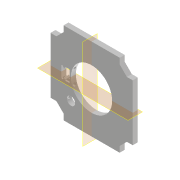
# Autodesk Inventor part: 20_Cube_Insert_lineartranlator_mgn7_base_v3
Saved by Autodesk Inventor 2022 (Build 260153000, 153)
## iProperties
Created: 2019-07-01
Part Number: 20_Cube_Insert_lineartranlator_mgn7_base_v3
Material: Generic
Document SubType Name: Modeling
Designer: diederichbenedict
Density: 1 g/cm^3
Appearance: Default
Author: diederichbenedict
Autodesk Inventor part; units mm, degrees
ref_plane "YZ Plane" through (0, 0, 0) normal (1, 0, 0) x (0, 1, 0)
ref_plane "XZ Plane" through (0, 0, 0) normal (0, 1, 0) x (-1, 0, 0)
ref_plane "Work Plane1" through (0, 0, 10) normal (0, 0, 1) x (1, 0, 0)
sketch "Sketch1" plane through (0, 0, 10) normal (0, 0, 1) x (1, 0, 0)
  line L0 (-4.0299, -0.3538) -> (-2.2322, 1.4439) construction
  arc A0 (-1.4439, 2.2322) -> (-2.2322, 1.4439) centre (-0.9299, 0.9299) ccw construction
  line L1 (-1.4439, 2.2322) -> (0.3538, 4.0299) construction
  line L2 (-37.8299, 42.8299) -> (-37.8299, 37.8299) construction
  line L3 (-37.8299, 37.8299) -> (-42.9208, 37.8299) construction
  line L4 (-37.8299, 42.2137) -> (-37.8299, 45.8299) construction
  line L5 (-37.8299, 45.8299) -> (-4.0299, 45.8299) construction
  line L6 (-4.0299, 45.8299) -> (-4.0299, 42.2137) construction
  line L7 (-4.0299, 4.0299) -> (0.3538, 4.0299) projected
  circle A1 centre (-20.9299, 20.9299) radius 17.5 projected
  line L8 (-20.9299, 58.9723) -> (17.1124, 20.9299) construction
  line L9 (17.1124, 20.9299) -> (-20.9299, -17.1124) construction
  line L10 (-20.9299, -17.1124) -> (-58.9723, 20.9299) construction
  line L11 (-58.9723, 20.9299) -> (-20.9299, 58.9723) construction
  line L12 (-20.9299, 58.9723) -> (-20.9299, -17.1124) construction
  line L13 (17.1124, 20.9299) -> (-58.9723, 20.9299) construction
  line L14 (-20.9299, 58.9723) -> (32.8701, 58.9723) construction
  line L15 (-43.4299, 43.4299) -> (1.5701, 43.4299) construction
  line L16 (1.5701, 43.4299) -> (1.5701, -1.5701) construction
  line L17 (1.5701, -1.5701) -> (-43.4299, -1.5701) construction
  line L18 (-43.4299, -1.5701) -> (-43.4299, 43.4299) construction
  line L19 (-43.4299, 43.4299) -> (1.5701, -1.5701) construction
  line L20 (1.5701, 43.4299) -> (-43.4299, -1.5701) construction
  line L21 (-43.4299, 5.3876) -> (-43.4299, 36.4723)
  line L22 (-43.4299, 36.4723) -> (-36.4723, 43.4299)
  line L23 (-36.4723, 43.4299) -> (-5.3876, 43.4299)
  line L24 (-5.3876, 43.4299) -> (1.5701, 36.4723)
  line L25 (1.5701, 36.4723) -> (1.5701, 5.3876)
  line L26 (1.5701, 5.3876) -> (-5.3876, -1.5701)
  line L27 (-5.3876, -1.5701) -> (-36.4723, -1.5701)
  line L28 (-36.4723, -1.5701) -> (-43.4299, 5.3876)
  line L29 (-4.0299, 42.2137) -> (-37.8299, 42.2137) projected
  line L30 (-4.0299, -0.3538) -> (-4.0299, 4.0299) projected
  circle A2 centre (-20.9299, 20.9299) radius 1.5
  line L31 (-10.9299, 10.9299) -> (-30.9299, 10.9299) construction
  line L32 (-30.9299, 10.9299) -> (-30.9299, 30.9299) construction
  line L33 (-30.9299, 30.9299) -> (-10.9299, 30.9299) construction
  line L34 (-10.9299, 30.9299) -> (-10.9299, 10.9299) construction
  line L35 (-10.9299, 10.9299) -> (-30.9299, 30.9299) construction
  line L36 (-30.9299, 10.9299) -> (-10.9299, 30.9299) construction
  circle A3 centre (-30.9299, 30.9299) radius 1.4
  circle A4 centre (-30.9299, 10.9299) radius 1.4
  circle A5 centre (-10.9299, 10.9299) radius 1.4
  line L37 (-45.8299, 37.8299) -> (-42.0723, 37.8299) construction
  line L38 (-42.1723, 37.7299) -> (-45.8299, 37.7299)
  line L39 (-45.8299, 37.7299) -> (-45.8299, 4.1299)
  line L40 (-45.8299, 4.1299) -> (-42.1723, 4.1299)
  line L41 (-42.1723, 4.1299) -> (-42.1723, 37.7299)
  line L42 (-45.8299, 4.0299) -> (-42.0723, 4.0299) construction
  line L43 (-45.8299, 37.8299) -> (-42.0723, 37.8299) projected
  line L44 (-37.7299, 45.8299) -> (-4.1299, 45.8299)
  line L45 (-4.1299, 45.8299) -> (-4.1299, 42.1723)
  line L46 (-4.1299, 42.1723) -> (-37.7299, 42.1723)
  line L47 (-37.7299, 42.1723) -> (-37.7299, 45.8299)
  line L48 (0.4701, 37.8299) -> (0.4701, 4.0299) construction
  line L49 (0.4701, 4.0299) -> (3.9701, 4.0299) construction
  line L50 (3.9701, 37.8299) -> (3.9701, 4.0299) construction
  line L51 (0.4701, 37.8299) -> (3.9701, 37.8299) construction
  line L52 (-45.8299, -3.9701) -> (-4.0299, -3.9701) construction
  line L53 (0.3124, 37.7299) -> (3.9701, 37.7299)
  line L54 (3.9701, 37.7299) -> (3.9701, 4.1299)
  line L55 (3.9701, 4.1299) -> (0.3124, 4.1299)
  line L56 (0.3124, 4.1299) -> (0.3124, 37.7299)
  line L57 (-4.1713, -0.3538) -> (-37.7299, -0.3538)
  line L58 (-37.7299, -0.3538) -> (-37.7299, -3.9701)
  line L59 (-37.7299, -3.9701) -> (-4.1713, -3.9701)
  line L60 (-4.1713, -3.9701) -> (-4.1713, -0.3538)
  point P0 (-37.8299, 4.0299)
  dimension "d18" = 53.8
  dimension "d19" = 45
  dimension "d20" = 53.8
  dimension "d21" = 45
  dimension "d22" = 45
  dimension "d30" = 20
  dimension "d31" = 20
  dimension "d32" = 2.8
  dimension "d33" = 2.8
  dimension "d34" = 2.8
  dimension "d35" = 3
  dimension "d36" = 0.1
  dimension "d37" = 0.1
  dimension "d38" = 0.1
  dimension "d39" = 0.1
  constraints: 86 end point, 21 point on line, 14 parallel, 8 perpendicular, 7 horizontal, 7 midpoint, 4 centre point, 4 coincident, 1 equal length
  measures "d18" distance of L8.start L8.end
  measures "d19" angle of L8 L14
  measures "d20" distance of L8.end L9.end
  measures "d21" distance of L16.end L17.end
  measures "d22" distance of L15.end L16.end
  measures "d30" distance of L32.end L33.end
  measures "d31" distance of L31.end L32.end
  measures "d32" diameter of A3
  measures "d33" diameter of A4
  measures "d34" diameter of A5
  measures "d35" diameter of A2
  measures "d36" distance between parallel lines of L38 L43
  measures "d37" distance between parallel lines of L40 L42
  measures "d38" distance between parallel lines of L45 L6
  measures "d39" distance between parallel lines of L4 L47
extrude "Extrusion1" add sketch "Sketch1" along normal blind 3 contours L30 L26 L57 L28 L41 L22 L46 L24 L56 L7 | L7 L26 L30 | L56 L24 L25 L26 | L26 L25 L24 L53 L54 L55 | L60 L59 L58 L57 L28 L27 L26 | L26 L27 L28 L57 | L46 L22 L29 L24 | L24 L29 L45 | L40 L39 L38 L22 L21 L28 | L28 L21 L22 L41 | L29 L22 L23 L24 | L24 L23 L22 L29 L47 L44 L45 | L47 L29 L22 | A1 | A2 | A3 | A4 | A5
sketch "Skizze4" plane through (0, 0, 13) normal (0, 0, 1) x (1, 0, 0)
  line L0 (-37.7299, 42.1723) -> (-42.1723, 37.7299) projected
  line L1 (-42.1723, 37.7299) -> (-45.8299, 37.7299) projected
  line L2 (-45.8299, 37.7299) -> (-45.8299, 4.1299) construction
  line L3 (-45.8299, 4.1299) -> (-42.1723, 4.1299) projected
  line L4 (-42.1723, 4.1299) -> (-37.6885, -0.3538) projected
  line L5 (-37.6885, -0.3538) -> (-37.7299, -0.3538) projected
  line L6 (-37.7299, -0.3538) -> (-37.7299, -3.9701) projected
  line L7 (-37.7299, -3.9701) -> (-4.1713, -3.9701) construction
  line L8 (-4.1713, -3.9701) -> (-4.1713, -0.3538) projected
  line L9 (-4.1713, -0.3538) -> (0.3124, 4.1299) projected
  line L10 (0.3124, 4.1299) -> (3.9701, 4.1299) projected
  line L11 (3.9701, 4.1299) -> (3.9701, 37.7299) construction
  line L12 (3.9701, 37.7299) -> (0.3124, 37.7299) projected
  line L13 (0.3124, 37.7299) -> (-4.1299, 42.1723) projected
  line L14 (-4.1299, 42.1723) -> (-4.1299, 45.8299) projected
  line L15 (-4.1299, 45.8299) -> (-37.7299, 45.8299) construction
  line L16 (-37.7299, 45.8299) -> (-37.7299, 42.1723) projected
  line L17 (-37.9299, 46.0299) -> (-3.9299, 46.0299) construction
  line L18 (-3.9299, 46.0299) -> (-3.9299, 42.2551)
  line L19 (-3.9299, 42.2551) -> (0.3953, 37.9299)
  line L20 (0.3953, 37.9299) -> (4.1701, 37.9299)
  line L21 (4.1701, 37.9299) -> (4.1701, 3.9299) construction
  line L22 (4.1701, 3.9299) -> (0.3953, 3.9299)
  line L23 (0.3953, 3.9299) -> (-3.9713, -0.4367)
  line L24 (-3.9713, -0.4367) -> (-3.9713, -4.1701)
  line L25 (-3.9713, -4.1701) -> (-37.9299, -4.1701) construction
  line L26 (-37.9299, -4.1701) -> (-37.9299, -0.3953)
  line L27 (-37.9299, -0.3953) -> (-42.2551, 3.9299)
  line L28 (-42.2551, 3.9299) -> (-46.0299, 3.9299)
  line L29 (-46.0299, 3.9299) -> (-46.0299, 37.9299) construction
  line L30 (-46.0299, 37.9299) -> (-42.2551, 37.9299)
  line L31 (-42.2551, 37.9299) -> (-37.9299, 42.2551)
  line L32 (-37.9299, 42.2551) -> (-37.9299, 46.0299)
  line L33 (-45.8299, 37.7299) -> (-45.8299, 37.9299)
  line L34 (-4.1299, 45.8299) -> (-37.7299, 45.8299) projected
  line L35 (-37.7299, 45.8299) -> (-37.9299, 45.8299)
  line L36 (-4.1299, 45.8299) -> (-3.9299, 45.8299)
  line L37 (3.9701, 37.7299) -> (3.9701, 37.9299)
  line L38 (3.9701, 4.1299) -> (3.9701, 37.7299) projected
  line L39 (3.9701, 4.1299) -> (3.9701, 3.9299)
  line L40 (-4.1713, -3.9701) -> (-3.9713, -3.9701)
  line L41 (-37.7299, -3.9701) -> (-37.9299, -3.9701)
  line L42 (-45.8299, 4.1299) -> (-45.8299, 3.9299)
  point P0 (0, 0)
  dimension "d40" = 0.2
  constraints: 48 end point, 12 point on line, 4 perpendicular, 15 other
  measures "d40" distance between parallel lines of L15 L17
extrude "IM_offset" add sketch "Skizze4" against normal up to surface (3 mm away)
ref_plane "Arbeitsebene5" through (-20.9299, 3.9299, 10) normal (1, 0, 0) x (0, 0, -1)
ref_plane "Arbeitsebene6" through (-37.9299, 20.9299, 10) normal (0, 1, 0) x (1, 0, 0)
sketch "Skizze25" plane through (0, 0, 13) normal (0, 0, 1) x (1, 0, 0)
  arc A0 (-37.9299, 18.0899) -> (-38.4737, 17.4299) centre (-37.6799, 17.3299) ccw projected
  line L0 (-37.9299, 18.0899) -> (-37.9299, 18.5899) projected
  line L1 (-37.9299, 18.5899) -> (-37.4299, 18.5899) projected
  line L2 (-37.4299, 18.5899) -> (-37.4299, 18.0899) projected
  arc A1 (-36.8862, 17.4299) -> (-37.4299, 18.0899) centre (-37.6799, 17.3299) ccw projected
  line L3 (-36.8862, 17.4299) -> (-34.5799, 17.4299) projected
  line L4 (-34.5799, 17.4299) -> (-34.3799, 17.6299) projected
  line L5 (-34.3799, 17.6299) -> (-34.3799, 24.2299) projected
  line L6 (-34.3799, 24.2299) -> (-34.5799, 24.4299) projected
  line L7 (-34.5799, 24.4299) -> (-36.8862, 24.4299) projected
  arc A2 (-37.4299, 23.77) -> (-36.8862, 24.4299) centre (-37.6799, 24.5299) ccw projected
  line L8 (-37.4299, 23.77) -> (-37.4299, 23.27) projected
  line L9 (-37.4299, 23.27) -> (-37.9299, 23.27) projected
  line L10 (-37.9299, 23.27) -> (-37.9299, 23.77) projected
  arc A3 (-38.4737, 24.4299) -> (-37.9299, 23.77) centre (-37.6799, 24.5299) ccw projected
  line L11 (-38.4737, 24.4299) -> (-38.9799, 24.4299) projected
  line L12 (-38.9799, 24.4299) -> (-39.1799, 24.2299) projected
  line L13 (-39.1799, 24.2299) -> (-39.1799, 17.6299) projected
  line L14 (-39.1799, 17.6299) -> (-38.9799, 17.4299) projected
  line L15 (-38.9799, 17.4299) -> (-38.4737, 17.4299) projected
  line L16 (-34.2799, 24.2713) -> (-34.2799, 17.5885)
  line L17 (-34.2799, 17.5885) -> (-34.5385, 17.3299)
  line L18 (-34.5385, 17.3299) -> (-36.9799, 17.3299)
  arc A4 (-36.9799, 17.3299) -> (-37.5299, 18.0137) centre (-37.6799, 17.3299) ccw
  line L19 (-37.5299, 18.0137) -> (-37.5299, 18.4899)
  line L20 (-37.5299, 18.4899) -> (-37.8299, 18.4899)
  line L21 (-37.8299, 18.4899) -> (-37.8299, 18.0137)
  arc A5 (-37.8299, 18.0137) -> (-38.3799, 17.3299) centre (-37.6799, 17.3299) ccw
  line L22 (-38.3799, 17.3299) -> (-39.0213, 17.3299)
  line L23 (-39.0213, 17.3299) -> (-39.2799, 17.5885)
  line L24 (-39.2799, 17.5885) -> (-39.2799, 24.2713)
  line L25 (-39.2799, 24.2713) -> (-39.0213, 24.5299)
  line L26 (-39.0213, 24.5299) -> (-38.3799, 24.5299)
  arc A6 (-38.3799, 24.5299) -> (-37.8299, 23.8462) centre (-37.6799, 24.5299) ccw
  line L27 (-37.8299, 23.8462) -> (-37.8299, 23.37)
  line L28 (-37.8299, 23.37) -> (-37.5299, 23.37)
  line L29 (-37.5299, 23.37) -> (-37.5299, 23.8462)
  arc A7 (-37.5299, 23.8462) -> (-36.9799, 24.5299) centre (-37.6799, 24.5299) ccw
  line L30 (-36.9799, 24.5299) -> (-34.5385, 24.5299)
  line L31 (-34.5385, 24.5299) -> (-34.2799, 24.2713)
  circle A8 centre (-21.0099, 20.9299) radius 10.125 projected
  circle A9 centre (-21.0099, 20.9299) radius 12.5
  point P0 (0, 0)
  dimension "d150" = 0.1
  dimension "d151" = 25
  constraints: 32 end point, 8 point on circle, 5 centre point, 1 coincident, 19 other
  measures "d150" distance between parallel lines of L5 L16
  measures "d151" diameter of A9
extrude "Extrusion21" cut sketch "Skizze25" against normal blind 3 contours A0 L15 L14 L13 L12 L11 A3 L10 L9 L8 A2 L7 L6 L5 L4 L3 A1 L2 L1 L0 | L16 L17 L18 A4 L19 L20 L21 A5 L22 L23 L24 L25 L26 A6 L27 L28 L29 A7 L30 L31 | A8 | A9
sketch "Skizze26" plane through (-45.8299, 3.9299, 10) normal (-1, 0, 0) x (0, 0, 1)
  line L0 (0, 0) -> (0, 34) projected
  line L1 (3, 0) -> (0, 0) projected
  line L2 (3, 34) -> (3, 0) projected
  line L3 (3, 34) -> (0, 34) projected
  line L4 (3, 29.5) -> (0, 29.5) projected
  circle A0 centre (1.5, 29.5) radius 0.9
  line L5 (3, 4.5) -> (0, 4.5) projected
  circle A1 centre (1.5, 4.5) radius 0.9
  line L6 (36.97, 20.3) -> (-3.03, 20.3) projected
  line L7 (36.97, 13.7) -> (-3.03, 13.7) projected
  circle A2 centre (1.5, 21.2) radius 0.9
  circle A3 centre (1.5, 12.8) radius 0.9
  point P0 (-10, -3.9299)
  dimension "d154" = 1.8
  dimension "d155" = 1.8
  dimension "d158" = 1.8
  dimension "d159" = 1.8
  constraints: 4 centre point, 2 midpoint, 2 tangent
  measures "d154" diameter of A0
  measures "d155" diameter of A1
  measures "d158" diameter of A2
  measures "d159" diameter of A3
extrude "Extrusion22" cut sketch "Skizze26" against normal blind 15 contours A3 | A1 L5 | L5 A1 | A2 | A0 L4 | L4 A0
sketch "Skizze27" plane through (0, 0, 10) normal (0, 0, -1) x (-1, 0, 0)
  arc A0 (36.9799, 24.5299) -> (37.5299, 23.8462) centre (37.6799, 24.5299) ccw projected
  line L0 (37.5299, 23.8462) -> (37.5299, 23.37) projected
  line L1 (37.5299, 23.37) -> (37.8299, 23.37) projected
  line L2 (37.8299, 23.37) -> (37.8299, 23.8462) projected
  arc A1 (37.8299, 23.8462) -> (38.3799, 24.5299) centre (37.6799, 24.5299) ccw projected
  line L3 (38.3799, 24.5299) -> (39.0213, 24.5299) projected
  line L4 (39.0213, 24.5299) -> (39.2799, 24.2713) projected
  line L5 (39.2799, 24.2713) -> (39.2799, 17.5885) projected
  line L6 (39.2799, 17.5885) -> (39.0213, 17.3299) projected
  line L7 (39.0213, 17.3299) -> (38.3799, 17.3299) projected
  arc A2 (38.3799, 17.3299) -> (37.8299, 18.0137) centre (37.6799, 17.3299) ccw projected
  line L8 (37.8299, 18.0137) -> (37.8299, 18.4899) projected
  line L9 (37.8299, 18.4899) -> (37.5299, 18.4899) projected
  line L10 (37.5299, 18.4899) -> (37.5299, 18.0137) projected
  arc A3 (37.5299, 18.0137) -> (36.9799, 17.3299) centre (37.6799, 17.3299) ccw projected
  line L11 (36.9799, 17.3299) -> (34.5385, 17.3299) projected
  line L12 (34.5385, 17.3299) -> (34.2799, 17.5885) projected
  line L13 (34.2799, 17.5885) -> (34.2799, 24.2713) projected
  line L14 (34.2799, 24.2713) -> (34.5385, 24.5299) projected
  line L15 (34.5385, 24.5299) -> (36.9799, 24.5299) projected
  circle A4 centre (21.0099, 20.9299) radius 12.5 projected
  line L16 (3.9713, -3.9701) -> (37.9299, -3.9701) projected
  line L17 (37.9299, -3.9701) -> (37.9299, -0.3953) projected
  line L18 (37.9299, -0.3953) -> (42.2551, 3.9299) projected
  line L19 (42.2551, 3.9299) -> (45.8299, 3.9299) projected
  line L20 (45.8299, 3.9299) -> (45.8299, 37.9299) projected
  line L21 (45.8299, 37.9299) -> (42.2551, 37.9299) projected
  line L22 (42.2551, 37.9299) -> (37.9299, 42.2551) projected
  line L23 (37.9299, 42.2551) -> (37.9299, 45.8299) projected
  line L24 (37.9299, 45.8299) -> (3.9299, 45.8299) projected
  line L25 (3.9299, 45.8299) -> (3.9299, 42.2551) projected
  line L26 (3.9299, 42.2551) -> (-0.3953, 37.9299) projected
  line L27 (-0.3953, 37.9299) -> (-3.9701, 37.9299) projected
  line L28 (-3.9701, 37.9299) -> (-3.9701, 3.9299) projected
  line L29 (-3.9701, 3.9299) -> (-0.3953, 3.9299) projected
  line L30 (-0.3953, 3.9299) -> (3.9713, -0.4367) projected
  line L31 (3.9713, -0.4367) -> (3.9713, -3.9701) projected
  line L32 (37.9799, 3.9599) -> (37.9799, 43.7799) projected
  line L33 (37.9799, 3.9599) -> (3.8799, 3.9599) projected
  circle A5 centre (33.4322, 8.4277) radius 3
  circle A6 centre (33.4322, 8.4277) radius 1.4
  point P0 (0, 0)
  point P1 (35.8514, 12.3014)
  dimension "d160" = 6
  constraints: 2 centre point, 3 other
  measures "d160" diameter of A5
extrude "Extrusion23" cut sketch "Skizze27" against normal blind 15 contours A5 | A6
body "Solid1"
